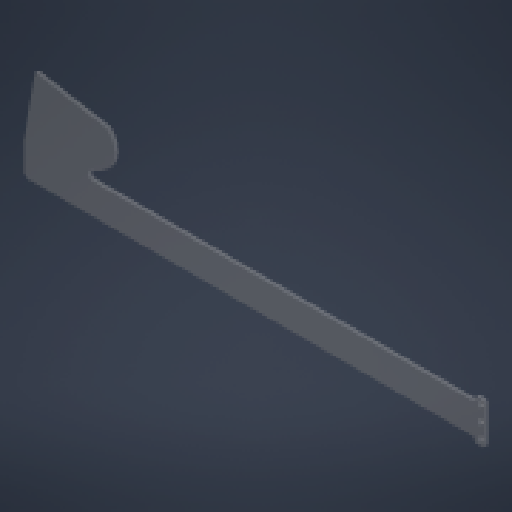
# Autodesk Inventor part: RACK_GUIDES
Saved by Autodesk Inventor 2026.2 (Build 302298010, 298A)
## iProperties
Created: 2026-04-01
Part Number: RACK_GUIDES
Material: Polycarbonate, PC 1000, Clear
Document SubType Name: Sheet Metal
Designer: 4aida
Density: 1.20131 g/cm^3
Sheet Metal Rule: Default
Appearance: Lexan (Clear)
Author: 4aida
Autodesk Inventor part; units mm, degrees
ref_plane "YZ Plane" through (0, 0, 0) normal (1, 0, 0) x (0, 1, 0)
ref_plane "XZ Plane" through (0, 0, 0) normal (0, 1, 0) x (-1, 0, 0)
ref_plane "XY Plane" through (0, 0, 0) normal (0, 0, 1) x (1, 0, 0)
sketch "Sketch1" plane through (0, 0, 0) normal (0, 0, 1) x (1, 0, 0)
  line L0 (279.4704, -19.05) -> (-282.4704, -19.05)
  line L1 (-282.4704, -19.05) -> (-282.4704, 19.05)
  line L2 (-282.4704, 19.05) -> (279.4704, 19.05)
  line L3 (282.4704, -19.05) -> (-282.4704, 19.05) construction
  line L4 (-282.4704, -19.05) -> (282.4704, 19.05) construction
  line L5 (292.1704, -25.05) -> (285.4704, -25.05)
  line L6 (285.4704, 25.05) -> (292.1704, 25.05)
  line L7 (295.1704, 22.05) -> (295.1704, -22.05)
  line L8 (295.1704, -25.05) -> (282.4704, 25.05) construction
  line L9 (282.4704, -25.05) -> (295.1704, 25.05) construction
  line L10 (282.4704, -22.05) -> (282.4704, -22.05)
  line L11 (282.4704, 22.05) -> (282.4704, 22.05)
  arc A0 (279.4704, 19.05) -> (282.4704, 22.05) centre (279.4704, 22.05) ccw
  arc A1 (285.4704, 25.05) -> (282.4704, 22.05) centre (285.4704, 22.05) ccw
  arc A2 (295.1704, 22.05) -> (292.1704, 25.05) centre (292.1704, 22.05) ccw
  arc A3 (292.1704, -25.05) -> (295.1704, -22.05) centre (292.1704, -22.05) ccw
  arc A4 (282.4704, -22.05) -> (285.4704, -25.05) centre (285.4704, -22.05) ccw
  arc A5 (282.4704, -22.05) -> (279.4704, -19.05) centre (279.4704, -22.05) ccw
  point P0 (0, 0)
  point P1 (288.8204, 0)
  point P2 (282.4704, 0)
  point P3 (295.1704, 0)
  dimension "d0" = 12.7
  dimension "d1" = 577.6407
  dimension "d2" = 6
  dimension "d3" = 38.1
  dimension "d4" = 3
  measures "d0" distance of L8.end L9.end
  measures "d1" distance between parallel lines of L7 L1
  measures "d2" distance between parallel lines of L2 L6
  measures "d3" distance between parallel lines of L2 L0
  measures "d4" radius of A0
extrude "Plate1" add sketch "Sketch1" along normal blind 4.7625
sketch "Sketch2" plane through (0, 0, 0) normal (0, 0, -1) x (-1, 0, 0)
  line L0 (-288.8204, -19.05) -> (-288.8204, 19.05)
  line L1 (-295.1704, -22.05) -> (-295.1704, 22.05) projected
  line L2 (-288.8204, 0) -> (-295.1704, 0)
  point P0 (0, 0)
  dimension "d6" = 6.35
  dimension "d7" = 38.1
  constraints: 4 end point, 2 midpoint, 1 coincident, 1 parallel, 1 perpendicular
  measures "d6" distance between parallel lines of L1 L0
  measures "d7" distance of L0.start L0.end
hole "Hole1" at (288.8204, -19.05, 0) at (288.8204, 0, 0) at (288.8204, 19.05, 0) direction (0, 0, 1) diameter 5.1054 depth 4.7625 tip angle 118 clearance for "Flat Head Machine Screw (82)" size "#10" standard "Ansi Unified Screw Threads"
sketch "Sketch3" plane through (0, 0, 0) normal (0, 0, -1) x (-1, 0, 0)
  line L0 (268.0066, 101.0778) -> (282.4704, 19.05)
  line L1 (180.2314, 85.6006) -> (268.0066, 101.0778)
  arc A0 (180.2314, 85.6006) -> (176.9524, 83.8547) centre (181.2732, 79.6918) ccw
  arc A1 (176.9524, 83.8547) -> (183.5568, 37.0593) centre (198.5568, 63.04) ccw
  line L2 (-279.4704, 19.05) -> (282.4704, 19.05)
  line L3 (282.4704, 19.05) -> (214.7497, 19.05)
  line L4 (282.4704, 19.05) -> (282.4704, -19.05)
  arc A2 (196.0756, 19.05) -> (196.0756, 31.05) centre (196.0756, 25.05) ccw
  line L5 (196.0756, 31.05) -> (193.9651, 31.05)
  line L6 (193.9651, 31.05) -> (183.5568, 37.0593)
  point P0 (0, 0)
  dimension "d16" = 43.99
  dimension "d17" = 80
  dimension "d18" = 83.9136
  dimension "d19" = 30
  dimension "d20" = 6
  dimension "d21" = 83.2932
  dimension "d28" = 12
  dimension "d29" = 86.3948
  dimension "d30" = 30
  measures "d16" distance from line of L2 A1.centre
  measures "d17" angle of L2 L0
  measures "d18" distance from line of L4 A1.centre
  measures "d19" radius of A1
  measures "d20" radius of A0
  measures "d21" distance from line of L0.end L1
  measures "d28" diameter of A2
  measures "d29" distance from line of L4 A2.centre
  measures "d30" angle of L2 L6
sheet face with bend "Face2" sketch "Sketch3" thickness 4.7625 toward (0, 0, 1) bend radius 4.7625 relief straight relief width 4.7625 relief depth 2.3813
bend "Bend1"
fillet "Corner Round1" radius 6.35 3 edges at (-282.4704, 19.05, 2.3813) (-282.4704, -19.05, 2.3813) (-193.9651, 31.05, 2.3813)
sketch "Sketch4" plane through (0, 0, 0) normal (0, 0, -1) x (-1, 0, 0)
  line L0 (268.0066, 101.0778) -> (180.2314, 85.6006) projected
  line L1 (282.3739, 19.5971) -> (268.0066, 101.0778) projected
  arc A0 (176.9524, 83.8547) -> (183.5568, 37.0593) centre (198.5568, 63.04) ccw projected
  circle A1 centre (198.5568, 63.04) radius 25.4
  line L2 (177.7503, 77.6089) -> (213.1256, 83.8465)
  line L3 (213.1256, 83.8465) -> (183.9879, 42.2336)
  line L4 (183.9879, 42.2336) -> (219.3632, 48.4712)
  line L5 (173.5426, 58.6294) -> (223.5709, 67.4507)
  point P0 (0, 0)
  point P1 (257.7049, 86.3654)
  point P2 (262.1156, 61.3512)
  dimension "d31" = 25.4
  dimension "d32" = 12.7
  dimension "d33" = 12.7
  dimension "d34" = 12.7
  dimension "d42" = 50.8
  dimension "d43" = 45
  constraints: 8 coincident, 8 end point, 6 point on circle, 3 parallel, 2 midpoint, 1 centre point
  measures "d31" distance of point (262.116, 61.351) point (257.705, 86.365)
  measures "d32" distance from line of L0 point (257.705, 86.365)
  measures "d33" distance from line of L1 point (257.705, 86.365)
  measures "d34" distance from line of L1 point (262.116, 61.351)
  measures "d42" diameter of A1
  measures "d43" angle of L2 L3
hole "Hole2" at (-257.7049, 86.3654, 0) at (-262.1156, 61.3512, 0) at (-177.7503, 77.6089, 0) at (-173.5426, 58.6294, 0) at (-183.9879, 42.2336, 0) at (-219.3632, 48.4712, 0) at (-223.5709, 67.4507, 0) at (-213.1256, 83.8465, 0) direction (0, 0, 1) diameter 5.105 end through all clearance for "Flat Head Machine Screw (82)" size "#10" standard "Ansi Unified Screw Threads"
equation "\"d13\" = Thickness"
equation "\"d33\" = d32"
equation "\"d34\" = d32"
equation "\"d40\" = Thickness"
equation "\"d5\" = Thickness"
equation "\"d22\" = BendRadius"
equation "\"d23\" = BendReliefWidth"
equation "\"d25\" = MinimumRemnant"
equation "\"d24\" = BendReliefDepth"
equation "\"d26\" = TransitionRadius"
equation "\"BendRadius\" = Thickness"
equation "\"BendReliefWidth\" = Thickness"
equation "\"BendReliefDepth\" = 0.5 * Thickness"
equation "\"CornerReliefSize\" = 4 * Thickness"
equation "\"MinimumRemnant\" = 2 * Thickness"
equation "\"TransitionRadius\" = BendRadius"
equation "\"JacobiRadiusSize\" = BendRadius"
equation "\"GapSize\" = Thickness"
equation "\"Thickness\" = 4.7625"
body "Solid1"
